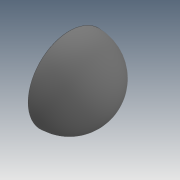
# Autodesk Inventor part: cover
Saved by Autodesk Inventor 2020.3 (Build 243373000, 373)
## iProperties
Created: 2021-01-25
Part Number: cover
Material: Generic
Document SubType Name: Modeling
Designer: serge
Density: 1 g/cm^3
Appearance: Gray
Author: serge
Autodesk Inventor part; units mm, degrees
ref_plane "YZ Plane" through (0, 0, 0) normal (1, 0, 0) x (0, 1, 0)
ref_plane "XZ Plane" through (0, 0, 0) normal (0, 1, 0) x (-1, 0, 0)
sketch "Sketch1" plane through (0, 0, 0) normal (1, 0, 0) x (0, 1, 0)
  circle A0 centre (0, 0) radius 25
  circle A1 centre (0, 0) radius 22
  line L0 (25, 0) -> (-25, 0)
  point P0 (-22, 0)
  point P1 (22, 0)
  dimension "d0" = 50
  dimension "d1" = 3
  constraints: 2 centre point, 2 coincident, 2 end point, 2 point on circle, 1 horizontal
  measures "d0" diameter of A0
  measures "d1" radial gap between concentric circles of A0 A1
revolve "Revolution1" add sketch "Sketch1" angle 360 about axis through (0, 25, 0) along (0, -1, 0) picked at (23.7578, -1.9943) contours A0 L0 A1
split "Split1" plane through (0, 0, 0) removes the side toward (-1, 0, 0)
sketch "Sketch2" plane through (0, 0, 0) normal (-1, 0, 0) x (0, 0, 1)
  line L0 (-13.5, -17.5) -> (13.5, -17.5)
  line L1 (13.5, -17.5) -> (13.5, 17.5)
  line L2 (13.5, 17.5) -> (-13.5, 17.5)
  line L3 (-13.5, 17.5) -> (-13.5, -17.5)
  line L4 (-13.5, -17.5) -> (13.5, 17.5) construction
  line L5 (13.5, -17.5) -> (-13.5, 17.5) construction
  line L6 (-15, -19) -> (15, -19)
  line L7 (15, -19) -> (15, 19)
  line L8 (15, 19) -> (-15, 19)
  line L9 (-15, 19) -> (-15, -19)
  line L10 (-15, -19) -> (15, 19) construction
  line L11 (15, -19) -> (-15, 19) construction
  point P0 (0, 0)
  dimension "d3" = 27
  dimension "d4" = 35
  dimension "d5" = 30
  dimension "d6" = 38
  constraints: 24 end point, 4 midpoint, 4 parallel, 2 horizontal, 2 perpendicular
  measures "d3" distance of L1.end L2.end
  measures "d4" distance of L2.end L0.start
  measures "d5" distance of L7.end L8.end
  measures "d6" distance of L8.end L6.start
extrude "Extrusion1" add sketch "Sketch2" against normal blind 6
ref_plane "Work Plane1" through (5, 0, 0) normal (-1, 0, 0) x (0, 0, 1)
sketch "Sketch3" plane through (5, 0, 0) normal (-1, 0, 0) x (0, 0, 1)
  line L0 (-13.481, -17.4685) -> (13.481, -17.4685)
  line L1 (13.481, -17.4685) -> (13.481, 17.4685)
  line L2 (13.481, 17.4685) -> (-13.481, 17.4685)
  line L3 (-13.481, 17.4685) -> (-13.481, -17.4685)
  line L4 (-13.481, -17.4685) -> (13.481, 17.4685) construction
  line L5 (13.481, -17.4685) -> (-13.481, 17.4685) construction
  line L6 (-13.481, 17.4685) -> (-6.481, 17.4685)
  line L7 (-6.481, 17.4685) -> (-6.481, 10.4685)
  line L8 (-6.481, 10.4685) -> (-13.481, 10.4685)
  line L9 (-13.481, 10.4685) -> (-13.481, 17.4685)
  line L10 (13.481, 17.4685) -> (6.481, 17.4685)
  line L11 (6.481, 17.4685) -> (6.481, 10.4685)
  line L12 (6.481, 10.4685) -> (13.481, 10.4685)
  line L13 (13.481, 10.4685) -> (13.481, 17.4685)
  line L14 (13.481, -17.4685) -> (6.481, -17.4685)
  line L15 (6.481, -17.4685) -> (6.481, -10.4685)
  line L16 (6.481, -10.4685) -> (13.481, -10.4685)
  line L17 (13.481, -10.4685) -> (13.481, -17.4685)
  line L18 (-13.481, -17.4685) -> (-6.481, -17.4685)
  line L19 (-6.481, -17.4685) -> (-6.481, -10.4685)
  line L20 (-6.481, -10.4685) -> (-13.481, -10.4685)
  line L21 (-13.481, -10.4685) -> (-13.481, -17.4685)
  point P0 (0, 0)
  point P1 (-13.481, 10.4685)
  point P2 (-6.481, 17.4685)
  point P3 (13.481, -10.4685)
  point P4 (13.481, 10.4685)
  point P5 (6.481, 17.4685)
  point P6 (-13.481, -10.4685)
  dimension "d10" = 34.937
  dimension "d11" = 26.9621
  dimension "d12" = 7
  dimension "d13" = 7
  dimension "d14" = 7
  dimension "d15" = 7
  dimension "d16" = 7
  dimension "d17" = 7
  dimension "d18" = 7
  dimension "d19" = 7
  constraints: 44 end point, 10 parallel, 5 horizontal, 5 perpendicular, 2 midpoint, 2 point on line
  measures "d10" distance of L0.end L1.end
  measures "d11" distance of L1.end L2.end
  measures "d12" distance of L11.end L12.end
  measures "d13" distance of L10.end L11.end
  measures "d14" distance of L7.end L8.end
  measures "d15" distance of L6.end L7.end
  measures "d16" distance of L19.end L20.end
  measures "d17" distance of L18.end L19.end
  measures "d18" distance of L14.end L15.end
  measures "d19" distance of L15.end L16.end
extrude "Extrusion2" add sketch "Sketch3" against normal up to next
sketch "Sketch4" plane through (0, 0, 0) normal (-1, 0, 0) x (0, 0, 1)
  line L0 (0, 0) -> (0, -25)
  circle A0 centre (0, 0) radius 25 projected
  line L1 (7, -17.5) -> (-7, -17.5)
  line L2 (-7, -17.5) -> (-7, -32.5)
  line L3 (-7, -32.5) -> (7, -32.5)
  line L4 (7, -32.5) -> (7, -17.5)
  line L5 (7, -17.5) -> (-7, -32.5) construction
  line L6 (-7, -17.5) -> (7, -32.5) construction
  dimension "d22" = 14
  dimension "d23" = 15
  constraints: 14 end point, 2 midpoint, 2 parallel, 1 horizontal, 1 perpendicular, 1 vertical, 1 vertical alignment, 1 other
  measures "d22" distance of L2.end L3.end
  measures "d23" distance of L3.end L1.start
extrude "Extrusion3" cut sketch "Sketch4" against normal blind 5 contours L1 L4 A0 L0 | L0 A0 L2 L1 | A0 L4 L3 L2
sketch "Sketch5" plane through (5, 0, 0) normal (-1, 0, 0) x (0, 0, 1)
  arc A0 (12.4037, -17.4685) -> (13.481, -16.6512) centre (0, 0) ccw projected
  line L0 (13.481, -16.6512) -> (13.481, 16.6512) projected
  line L1 (-12.4037, -17.4685) -> (12.4037, -17.4685) projected
  arc A1 (13.481, 16.6512) -> (12.4037, 17.4685) centre (0, 0) ccw projected
  line L2 (12.4037, 17.4685) -> (-12.4037, 17.4685) projected
  line L3 (13.481, -16.6512) -> (13.481, 16.6512) projected
  arc A2 (-12.4037, 17.4685) -> (-13.481, 16.6512) centre (0, 0) ccw projected
  line L4 (-13.481, 16.6512) -> (-13.481, -16.6512) projected
  line L5 (12.4037, 17.4685) -> (-12.4037, 17.4685) projected
  arc A3 (-13.481, -16.6512) -> (-12.4037, -17.4685) centre (0, 0) ccw projected
  line L6 (-12.4037, -17.4685) -> (12.4037, -17.4685) projected
  line L7 (-13.481, 16.6512) -> (-13.481, -16.6512) projected
  line L8 (-9.75, -12.4685) -> (9.75, -12.4685) construction
  line L9 (9.75, -12.4685) -> (9.75, 13.5315) construction
  line L10 (9.75, 13.5315) -> (-9.75, 13.5315) construction
  line L11 (-9.75, 13.5315) -> (-9.75, -12.4685) construction
  line L12 (-9.75, -12.4685) -> (9.75, 13.5315) construction
  line L13 (9.75, -12.4685) -> (-9.75, 13.5315) construction
  circle A4 centre (-9.75, 13.5315) radius 0.875
  circle A5 centre (-9.75, -12.4685) radius 0.875
  arc A6 (12.4037, -17.4685) -> (13.481, -16.6512) centre (0, 0) ccw projected
  line L14 (13.481, -16.6512) -> (13.481, 16.6512) projected
  arc A7 (13.481, 16.6512) -> (12.4037, 17.4685) centre (0, 0) ccw projected
  line L15 (12.4037, 17.4685) -> (-12.4037, 17.4685) projected
  arc A8 (-12.4037, 17.4685) -> (-13.481, 16.6512) centre (0, 0) ccw projected
  arc A9 (-13.481, -16.6512) -> (-12.4037, -17.4685) centre (0, 0) ccw projected
  line L16 (-12.4037, -17.4685) -> (12.4037, -17.4685) projected
  arc A10 (12.4037, -17.4685) -> (13.481, -16.6512) centre (0, 0) ccw projected
  line L17 (13.481, -16.6512) -> (13.481, 16.6512) projected
  arc A11 (13.481, 16.6512) -> (12.4037, 17.4685) centre (0, 0) ccw projected
  arc A12 (-13.481, -16.6512) -> (-12.4037, -17.4685) centre (0, 0) ccw projected
  line L18 (-12.4037, -17.4685) -> (12.4037, -17.4685) projected
  arc A13 (12.4037, -17.4685) -> (13.481, -16.6512) centre (0, 0) ccw projected
  arc A14 (-12.4037, 17.4685) -> (-13.481, 16.6512) centre (0, 0) ccw projected
  line L19 (-13.481, 16.6512) -> (-13.481, -16.6512) projected
  arc A15 (-13.481, -16.6512) -> (-12.4037, -17.4685) centre (0, 0) ccw projected
  arc A16 (13.481, 16.6512) -> (12.4037, 17.4685) centre (0, 0) ccw projected
  line L20 (12.4037, 17.4685) -> (-12.4037, 17.4685) projected
  arc A17 (-12.4037, 17.4685) -> (-13.481, 16.6512) centre (0, 0) ccw projected
  line L21 (-13.481, 16.6512) -> (-13.481, -16.6512) projected
  line L22 (-12.4037, -17.4685) -> (12.4037, -17.4685) projected
  line L23 (0, -17.4685) -> (0, -12.4685)
  line L24 (0, -12.4685) -> (9.75, -12.4685)
  dimension "d50" = 19.5
  dimension "d51" = 26
  dimension "d52" = 1.75
  dimension "d53" = 1.75
  dimension "d64" = 5
  constraints: 16 end point, 2 centre point, 2 coincident, 2 horizontal, 2 parallel, 1 perpendicular, 1 vertical, 2 other
  measures "d50" distance of L9.end L10.end
  measures "d51" distance of L10.end L8.start
  measures "d52" diameter of A4
  measures "d53" diameter of A5
  measures "d64" distance of L23.start L23.end
sketch "Sketch6" plane through (0, -17.371, -13.5) normal (-1, 0, 0) x (0, 0, 1)
  line L0 (27.5, -0.629) -> (-0.5, -0.629)
  line L1 (-0.5, -0.629) -> (-0.5, 35.371)
  line L2 (-0.5, 35.371) -> (27.5, 35.371)
  line L3 (27.5, 35.371) -> (27.5, -0.629)
  line L4 (27.5, -0.629) -> (-0.5, 35.371) construction
  line L5 (-0.5, -0.629) -> (27.5, 35.371) construction
  point P0 (13.5, 17.371)
  dimension "d30" = 36
  dimension "d31" = 28
  constraints: 12 end point, 2 midpoint, 2 parallel, 1 horizontal, 1 perpendicular
  measures "d30" distance of L0.end L1.end
  measures "d31" distance of L0.start L0.end
extrude "Extrusion5" cut sketch "Sketch6" against normal blind 4.5
sketch "Sketch7" plane through (0, -19, 7) normal (-1, 0, 0) x (0, 0, 1)
  line L0 (8, 33.9332) -> (8, 4.0668) projected
  line L1 (8, 19) -> (15, 19)
  arc A0 (8, 2.9065) -> (8, 35.0935) centre (-7, 19) ccw projected
  line L2 (15, 20) -> (8, 20)
  line L3 (8, 20) -> (8, 18)
  line L4 (8, 18) -> (15, 18)
  line L5 (15, 18) -> (15, 20)
  line L6 (15, 20) -> (8, 18) construction
  line L7 (8, 20) -> (15, 18) construction
  point P0 (11.5, 19)
  point P1 (14.9773, 20)
  point P2 (8, 20)
  point P3 (14.9773, 18)
  dimension "d34" = 2
  constraints: 14 end point, 4 midpoint, 2 horizontal, 2 parallel, 1 perpendicular, 1 point on circle, 1 point on line
  measures "d34" distance of L4.end L2.start
extrude "Extrusion6" add sketch "Sketch7" against normal blind 2 contours L2 A0 L1 L0 | L1 A0 L4 L0
pattern_linear "Rectangular Pattern1" count 3 spacing 10 along (0, -1, 0) of "Extrusion6" first direction both ways yes
mirror "Mirror3" about plane through (0, 0, 0) normal (0, 0, 1) of "Extrusion6", "Rectangular Pattern1"
sketch "Sketch8" plane through (0, -19, 7) normal (-1, 0, 0) x (0, 0, 1)
  circle A0 centre (-7, 19) radius 24.125
  circle A1 centre (-7, 19) radius 22.875
  dimension "d40" = 48.25
  dimension "d41" = 1.25
  constraints: 2 centre point, 2 coincident
  measures "d40" diameter of A0
  measures "d41" radial gap between concentric circles of A0 A1
extrude "Extrusion7" cut sketch "Sketch8" against normal blind 3.5
extrude "Extrusion8" cut sketch "Sketch5" against normal blind 7.5 contours A4 | A5
mirror "Mirror4" about plane through (0, 0, 0) normal (0, 0, 1) of "Extrusion8"
sketch "Sketch10" plane through (5, 0, 0) normal (-1, 0, 0) x (0, 0, 1)
  line L0 (-8, -14) -> (8, -14)
  line L1 (8, -14) -> (8, 14)
  line L2 (8, 14) -> (-8, 14)
  line L3 (-8, 14) -> (-8, -14)
  line L4 (-8, -14) -> (8, 14) construction
  line L5 (8, -14) -> (-8, 14) construction
  line L6 (-13, -11) -> (13, -11)
  line L7 (13, -11) -> (13, 11)
  line L8 (13, 11) -> (-13, 11)
  line L9 (-13, 11) -> (-13, -11)
  line L10 (-13, -11) -> (13, 11) construction
  line L11 (13, -11) -> (-13, 11) construction
  point P0 (0, 0)
  point P1 (-8, 11)
  point P2 (-8, -11)
  point P3 (8, -11)
  point P4 (8, 11)
  dimension "d67" = 16
  dimension "d68" = 22
  dimension "d69" = 28
  dimension "d70" = 26
  constraints: 24 end point, 4 midpoint, 4 parallel, 2 horizontal, 2 perpendicular
  measures "d67" distance of L1.end L2.end
  measures "d68" distance of L8.end L6.start
  measures "d69" distance of L2.end L0.start
  measures "d70" distance of L7.end L8.end
extrude "Extrusion10" cut sketch "Sketch10" against normal blind 10
fillet "Fillet3" radius 2 4 edges at (10, 11, -8) (10, 11, 8) (10, -11, -8) (10, -11, 8)
fillet "Fillet4" radius 2 4 edges at (10, 14, -8) (10, 14, 8) (10, -14, -8) (10, -14, 8)
sketch "Sketch11" plane through (0, -19, -11.0905) normal (-1, 0, 0) x (0, 0, 1)
  line L0 (11.2667, 37.0291) -> (11.2667, 40.9993) construction
  arc A0 (22.1811, 38) -> (0, 38) centre (11.0905, 19) ccw projected
  line L1 (-2.9095, 37) -> (25.0905, 37) projected
  line L2 (10.2667, 41.0284) -> (12.2667, 41.0284)
  line L3 (12.2667, 41.0284) -> (12.2667, 37)
  line L4 (12.2667, 37) -> (10.2667, 37)
  line L5 (10.2667, 37) -> (10.2667, 41.0284)
  line L6 (10.2667, 41.0284) -> (12.2667, 37) construction
  line L7 (12.2667, 41.0284) -> (10.2667, 37) construction
  point P0 (11.2667, 39.0142)
  point P1 (10.2667, 40.9846)
  point P2 (12.2667, 40.9685)
  dimension "d75" = 2
  constraints: 14 end point, 3 midpoint, 2 parallel, 1 horizontal, 1 perpendicular, 1 point on circle, 1 point on line, 1 vertical
  measures "d75" distance between parallel lines of L5 L3
extrude "Extrusion11" add sketch "Sketch11" against normal blind 10 contours L3 L1 L5 A0
body "Solid1"
